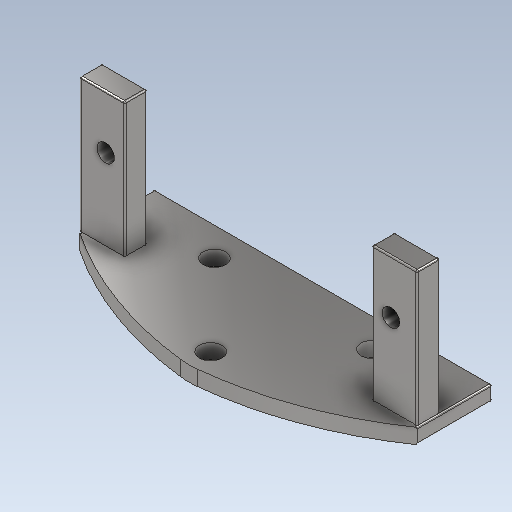
# Autodesk Inventor part: holder
Saved by Autodesk Inventor 2020 (Build 240168000, 168)
## iProperties
Created: 2020-05-08
Part Number: holder
Material: Сталь, нержавеющая, аустенитная
Document SubType Name: Modeling
Designer: jamnissa
Density: 8 g/cm^3
Appearance: С умеренной полировкой
Mass: 15.4465 g
Surface Area: 22.5297 cm^2
Volume: 1.93081 cm^3
Author: jamnissa
Autodesk Inventor part; units mm, degrees
ref_plane "YZ Plane" through (0, 0, 0) normal (1, 0, 0) x (0, 1, 0)
sketch "Эскиз1" plane through (0, 0, 0) normal (0, 0, 1) x (1, 0, 0)
  circle A0 centre (2.5, 13.5) radius 4.7
  circle A1 centre (12.5, 13.5) radius 5.2
  line L0 (10.7517, 6) -> (21, 6)
  arc A2 (21, 6) -> (24, 9) centre (21, 9) ccw
  line L1 (24, 9) -> (24, 18)
  arc A3 (24, 18) -> (21, 21) centre (21, 18) ccw
  line L2 (21, 21) -> (-6, 21)
  arc A4 (-6, 21) -> (-9, 18) centre (-6, 18) ccw
  line L3 (-9, 18) -> (-9, 9)
  arc A5 (-9, 9) -> (-6, 6) centre (-6, 9) ccw
  line L4 (-6, 6) -> (3.8468, 6)
  line L5 (3.8468, 7.8329) -> (3.8468, 6)
  line L6 (10.7517, 7.8329) -> (3.8468, 7.8329)
  line L7 (10.7517, 6) -> (10.7517, 7.8329)
  arc A6 (7.2375, 11.9012) -> (7.2375, 15.0988) centre (12.5, 13.5) ccw
  arc A7 (7.2375, 15.0988) -> (7.2375, 11.9012) centre (2.5, 13.5) ccw
  circle A8 centre (-6, 18) radius 0.6
  circle A9 centre (21, 18) radius 0.6
  circle A10 centre (21, 9) radius 0.6
  circle A11 centre (-6, 9) radius 0.6
  circle A12 centre (-6, 18) radius 0.6
  line L8 (10.7517, 6) -> (21, 6)
  arc A13 (21, 6) -> (24, 9) centre (21, 9) ccw
  line L9 (24, 9) -> (24, 18)
  arc A14 (24, 18) -> (21, 21) centre (21, 18) ccw
  line L10 (21, 21) -> (-6, 21)
  arc A15 (-6, 21) -> (-9, 18) centre (-6, 18) ccw
  line L11 (-9, 18) -> (-9, 9)
  arc A16 (-9, 9) -> (-6, 6) centre (-6, 9) ccw
  line L12 (-6, 6) -> (3.8468, 6)
  line L13 (3.8468, 7.8329) -> (3.8468, 6)
  line L14 (10.7517, 7.8329) -> (3.8468, 7.8329)
  line L15 (10.7517, 6) -> (10.7517, 7.8329)
  arc A17 (7.2375, 11.9012) -> (7.2375, 15.0988) centre (12.5, 13.5) ccw
  arc A18 (7.2375, 15.0988) -> (7.2375, 11.9012) centre (2.5, 13.5) ccw
  circle A19 centre (-6, 18) radius 0.6
  circle A20 centre (21, 18) radius 0.6
  circle A21 centre (21, 9) radius 0.6
  circle A22 centre (-6, 9) radius 0.6
  arc A23 (7.2375, 15.0988) -> (7.2375, 11.9012) centre (2.5, 13.5) ccw
  arc A24 (7.2375, 11.9012) -> (7.2375, 15.0988) centre (12.5, 13.5) ccw
  circle A25 centre (21, 18) radius 0.6
  circle A26 centre (21, 9) radius 0.6
  circle A27 centre (26.4592, 13.9084) radius 1.175
  line L16 (27.8433, 16.57) -> (23.9394, 18.6)
  arc A28 (28.2111, 11.473) -> (27.8433, 16.57) centre (26.4592, 13.9084) ccw
  line L17 (23.9394, 8.4) -> (28.2111, 11.473)
  line L18 (24, 9) -> (24, 18)
  line L19 (-9, 18) -> (-9, 9)
  line L20 (-12.8433, 16.57) -> (-8.9394, 18.6)
  arc A29 (-12.8433, 16.57) -> (-13.2111, 11.473) centre (-11.4592, 13.9084) ccw
  line L21 (-8.9394, 8.4) -> (-13.2111, 11.473)
  circle A30 centre (-11.4592, 13.9084) radius 1.175
  line L22 (10.7517, 7.8329) -> (3.8468, 7.8329)
  line L23 (3.8468, 7.8329) -> (3.8468, 6)
  line L24 (10.7517, 6) -> (10.7517, 7.8329)
  line L25 (3.8468, 6) -> (10.7517, 6)
  line L26 (-8.9394, 3) -> (-14.9394, 3)
  line L27 (-14.9394, 3) -> (-14.9394, 21)
  line L28 (-14.9394, 21) -> (-8.9394, 21)
  line L29 (-8.9394, 21) -> (-8.9394, 3)
  line L30 (29.9364, 3) -> (23.9364, 3)
  line L31 (23.9364, 3) -> (23.9364, 21)
  line L32 (23.9364, 21) -> (29.9364, 21)
  line L33 (29.9364, 21) -> (29.9364, 3)
  point P0 (0, 0)
  point P1 (7.5, 13.5)
  dimension "d1" = 6
  dimension "d2" = 18
  dimension "d3" = 6
  dimension "d4" = 18
  constraints: 68 end point, 32 point on circle, 31 centre point, 4 parallel, 2 horizontal, 2 perpendicular
  measures "d1" distance of L27.end L28.end
  measures "d2" distance of L26.end L27.end
  measures "d3" distance of L31.end L32.end
  measures "d4" distance of L31.start L31.end
extrude "Выдавливание1" add sketch "Эскиз1" against normal blind 3 contours L31 A3 L1 A2 | A2 L17 A28 L16 A3 L31 L32 L33 L30 | A2 L1 A3 L16 A28 L17 | L21 A29 L20 A4 L3 A5 | L29 L26 L27 L28 L20 A29 L21 | A5 L3 A4 L29 | A27 | A30
fillet "Сопряжение1" radius 0.2 24 edges at (26.9364, 21, 0) (29.9364, 12, 0) (23.9364, 12, 0) (23.9364, 21, -1.5) (23.9364, 12, -3) (23.9364, 3, -1.5) (26.9364, 3, 0) (26.9364, 3, -3) (29.9364, 3, -1.5) (29.9364, 12, -3) (29.9364, 21, -1.5) (26.9364, 21, -3) (-11.9394, 3, 0) (-14.9394, 3, -1.5) (-11.9394, 3, -3) (-8.9394, 3, -1.5) (-8.9394, 12, 0) (-8.9394, 12, -3) (-8.9394, 21, -1.5) (-11.9394, 21, 0) (-11.9394, 21, -3) (-14.9394, 21, -1.5) (-14.9394, 12, 0) (-14.9394, 12, -3)
ref_plane "РабПлоскость1" through (-11.9394, 3, -0.2) normal (0, -1, 0) x (1, 0, 0)
sketch "Эскиз2" plane through (-11.9394, 3, -0.2) normal (0, -1, 0) x (1, 0, 0)
  line L0 (41.8758, -2.6) -> (41.8758, 0) projected
  arc A0 (41.6758, -2.8) -> (41.8758, -2.6) centre (41.6758, -2.6) ccw projected
  line L1 (36.0758, -2.8) -> (41.6758, -2.8) projected
  arc A1 (35.8758, -2.6) -> (36.0758, -2.8) centre (36.0758, -2.6) ccw projected
  line L2 (35.8758, 0) -> (35.8758, -2.6) projected
  arc A2 (41.8758, 0) -> (41.6758, 0.2) centre (41.6758, 0) ccw projected
  line L3 (41.8758, 0.2) -> (35.8758, 0.2) projected
  arc A3 (36.0758, 0.2) -> (35.8758, 0) centre (36.0758, 0) ccw projected
  line L4 (-2.8, -2.8) -> (2.8, -2.8) projected
  arc A4 (2.8, -2.8) -> (3, -2.6) centre (2.8, -2.6) ccw projected
  line L5 (3, -2.6) -> (3, 0) projected
  line L6 (-3, 0) -> (-3, -2.6) projected
  arc A5 (-3, -2.6) -> (-2.8, -2.8) centre (-2.8, -2.6) ccw projected
  arc A6 (-2.8, 0.2) -> (-3, 0) centre (-2.8, 0) ccw projected
  arc A7 (3, 0) -> (2.8, 0.2) centre (2.8, 0) ccw projected
  line L7 (3, 0.2) -> (-3, 0.2) projected
  line L8 (41.8758, 0.2) -> (-3, 0.2)
  line L9 (-3, 0.2) -> (-3, -9.8)
  line L10 (-3, -9.8) -> (41.8758, -9.8)
  line L11 (41.8758, -9.8) -> (41.8758, 0.2)
  line L12 (19.4379, -15.6542) -> (19.4379, 4.8221)
  circle A8 centre (29.9379, -5.8) radius 1.5
  circle A9 centre (8.9379, -5.8) radius 1.5
  line L13 (19.4379, 0.2) -> (19.4379, 10.2)
  line L14 (19.4379, 0.2) -> (19.4379, -44.8)
  circle A10 centre (19.4379, -44.8) radius 55
  circle A11 centre (19.4379, -44.8) radius 50
  circle A12 centre (19.4379, 5.2) radius 1.5
  circle A13 centre (19.4379, 5.2) radius 3
  arc A14 (19.4379, 8.2) -> (-3, 0.2) centre (23.8819, -39.7303) ccw
  arc A15 (41.8758, 0.2) -> (19.4379, 8.2) centre (15.7571, -37.5899) ccw
  point P0 (11.9394, 0.2)
  point P1 (41.8758, 0)
  point P2 (0, 0)
  point P3 (0, 0)
  dimension "d53" = 100
  dimension "d55" = 6
  dimension "d14" = 3
  dimension "d15" = 3
  dimension "d17" = 21
  dimension "d19" = 10
  dimension "d20" = 4
  dimension "d49" = 10
  dimension "d50" = 45
  dimension "d51" = 110
  dimension "d54" = 3
  constraints: 14 end point, 6 centre point, 4 point on circle, 4 point on line, 4 vertical, 3 coincident, 2 midpoint, 2 vertical alignment, 1 perpendicular, 1 symmetric about line, 4 other
  measures "d14" diameter of A8
  measures "d15" diameter of A9
  measures "d17" distance of A9.centre A8.centre
  measures "d19" distance of L8.end L9.end
  measures "d20" distance from line of L10 A8.centre
  measures "d49" distance of L13.start L13.end
  measures "d50" distance of L13.start L14.end
  measures "d51" diameter of A10
  measures "d54" diameter of A12
extrude "Выдавливание2" add sketch "Эскиз2" along normal blind 2 contours A0 L1 A1 L2 A3 L3 A11 L0 | L11 L10 L12 L8 L3 A3 L2 A1 L1 A0 | A11 L3 A2 L0 | A2 L3 L11 | A11 A13 A15 L3 | L3 L8 L12 A13 A11 | L10 L9 A5 L4 A4 L5 A7 L7 L8 L12 | A11 L7 A7 L5 A4 L4 A5 L6 | L6 A6 L7 A11 | A13 L12 A12 A11 | A11 A12 L13 A15 A13 | L8 L7 A11 A13 L12 | L9 L7 A6 | L7 A14 A13 A11 | A12 L12 L13 A11 | A11 L13 A12 | A13 A11 A12 L12 | L13 A12 A11 A13 A14 | A11 A12 L13 | L13 L12 A12 A11 | A8 | A9
extrude "Выдавливание3" cut sketch "Эскиз2" along normal through all contours A12 L12 L13 A11 | A11 L13 A12 | A11 A12 L13 | L13 L12 A12 A11 | A8 | A9
fillet "Сопряжение2" radius 0.2 8 edges at (29.9364, 3, -5) (7.4985, 3, -10) (-14.9394, 3, -5) (29.9364, 1, -5) (29.9364, 2, -10) (7.4985, 1, -10) (-14.9394, 2, -10) (-14.9394, 1, -5)
extrude "Выдавливание4" cut sketch "Эскиз1" against normal through all contours A27 | A30
fillet "Сопряжение3" radius 10 1 edges at (7.4985, 2, 8)
ref_plane "РабПлоскость2" through (-11.9394, 2, -0.2) normal (0, 1, 0) x (1, 0, 0)
sketch "Эскиз3" plane through (-11.9394, 2, -0.2) normal (0, 1, 0) x (1, 0, 0)
  circle A0 centre (19.4379, -5.2) radius 1.5 projected
  circle A1 centre (8.9379, 5.8) radius 1.5 projected
  circle A2 centre (29.9379, 5.8) radius 1.5 projected
  point P0 (11.9394, -0.2)
